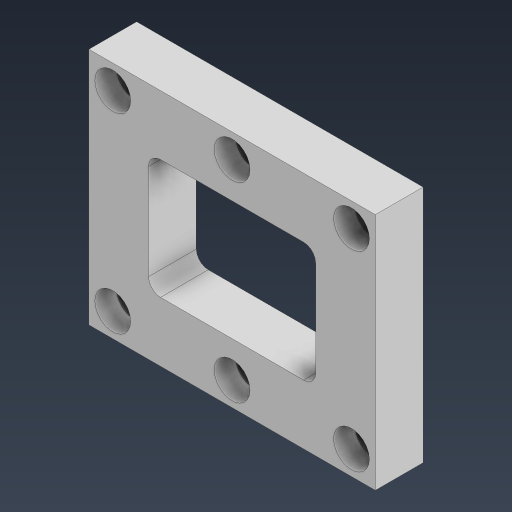
# Autodesk Inventor part: 3D Model
Saved by Autodesk Inventor 2024 (Build 280153000, 153)
## iProperties
Created: 2024-03-13
Part Number: 3D Model
Material: Genérico
Document SubType Name: Modeling
Designer: Administrator
Density: 1 g/cm^3
Appearance: Padrão
Author: Administrator
Autodesk Inventor part; units mm, degrees
ref_plane "YZ Plane" through (0, 0, 0) normal (1, 0, 0) x (0, 1, 0)
ref_plane "XZ Plane" through (0, 0, 0) normal (0, 1, 0) x (-1, 0, 0)
ref_plane "XY Plane" through (0, 0, 0) normal (0, 0, 1) x (1, 0, 0)
sketch "Esboço1" plane through (0, 0, 0) normal (0, 0, 1) x (1, 0, 0)
  line L0 (-60, -50) -> (60, -50)
  line L1 (60, -50) -> (60, 50)
  line L2 (60, 50) -> (-60, 50)
  line L3 (-60, 50) -> (-60, -50)
  line L4 (-60, -50) -> (60, 50) construction
  line L5 (60, -50) -> (-60, 50) construction
  line L6 (-35, 25) -> (35, 25)
  line L7 (35, 25) -> (35, -25)
  line L8 (35, -25) -> (-35, -25)
  line L9 (-35, -25) -> (-35, 25)
  line L10 (-35, 25) -> (35, -25) construction
  line L11 (35, 25) -> (-35, -25) construction
  point P0 (0, 0)
  dimension "d0" = 120
  dimension "d1" = 100
  dimension "d2" = 70
  dimension "d3" = 50
  constraints: 24 end point, 4 midpoint, 4 parallel, 2 horizontal, 2 perpendicular
  measures "d0" distance of L2.end L1.end
  measures "d1" distance of L1.end L0.end
  measures "d2" distance of L7.end L8.end
  measures "d3" distance of L6.end L7.end
extrude "Extrusão1" add sketch "Esboço1" along normal blind 20
fillet "Arredondamento1" radius 5 4 edges at (-35, 25, 10) (35, 25, 10) (-35, -25, 10) (35, -25, 10)
sketch "Esboço2" plane through (0, 0, 20) normal (0, 0, 1) x (1, 0, 0)
  line L0 (-60, 50) -> (-60, -50) projected
  line L1 (60, 50) -> (-60, 50) projected
  point P0 (0, 0)
  point P1 (-50, 40)
  dimension "d14" = 10
  dimension "d15" = 10
  measures "d14" distance from line of L0 point (-50, 40)
  measures "d15" distance from line of L1 point (-50, 40)
hole "Furo1" at (-50, 40, 20) direction (0, 0, -1) diameter 9 end through all counterbore diameter 15 counterbore depth 9
pattern_linear "Padrão retangular1" count 2 spacing 80 along (0, -1, 0) count 3 spacing 50 along (1, 0, 0) of "Furo1"
